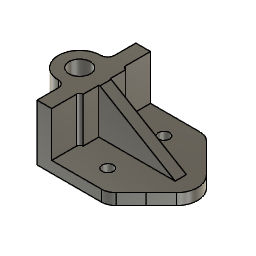
A3 (Autodesk Fusion 360 design; units mm, degrees)
Autodesk Fusion 360 part; units mm, degrees
sketch "BaseA3" plane through (0, 0, 0) normal (0, 0, 1) x (1, 0, 0)
  line L0 (0, 0) -> (28, 0)
  line L1 (28, 88) -> (0, 88)
  line L2 (0, 0) -> (-3, 0)
  line L3 (-3, 88) -> (0, 88)
  line L4 (-3, 0) -> (-16, 0)
  line L5 (-16, 88) -> (-3, 88)
  line L6 (-9.5, 0) -> (-9.5, 44) construction
  line L7 (-9.5, 44) -> (-16, 44) construction
  line L8 (-16, 44) -> (-22, 44) construction
  circle A0 centre (-22, 44) radius 9.5
  arc A1 (-22, 63) -> (-22, 25) centre (-22, 44) ccw
  line L9 (-16, 0) -> (-16, 19)
  line L10 (-16, 69) -> (-16, 88)
  arc A2 (-22, 63) -> (-16, 69) centre (-22, 69) ccw
  arc A3 (-16, 19) -> (-22, 25) centre (-22, 19) ccw
  line L11 (0, 63) -> (0, 63)
  line L12 (0, 25) -> (0, 22) construction
  line L13 (0, 22) -> (-3, 22) construction
  arc A4 (0, 25) -> (-3, 22) centre (0, 22) ccw
  line L14 (-9.5, 44) -> (0, 44) construction
  arc A5 (-3, 66) -> (0, 63) centre (0, 66) ccw
  line L15 (-22, 69) -> (-22, 63) construction
  line L16 (-22, 69) -> (-16, 69) construction
  line L17 (-22, 63) -> (-22, 25) construction
  line L18 (-22, 25) -> (-22, 19) construction
  line L19 (-22, 19) -> (-16, 19) construction
  line L20 (0, 63) -> (0, 66) construction
  line L21 (0, 66) -> (-3, 66) construction
  line L22 (-3, 69) -> (28, 69) construction
  circle A6 centre (28, 69) radius 5
  line L23 (0, 44) -> (28, 44) construction
  circle A7 centre (28, 19) radius 5
  line L24 (-3, 19) -> (28, 19) construction
  line L25 (28, 19) -> (64, 19) construction
  line L26 (64, 19) -> (64, 69) construction
  line L27 (64, 69) -> (28, 69) construction
  line L28 (28, 0) -> (46.834, 0)
  line L29 (46.834, 0) -> (64, 17.146)
  line L30 (64, 17.146) -> (77.427, 30.5569)
  line L31 (28, 44) -> (83, 44) construction
  line L32 (64, 70.854) -> (77.427, 57.4431)
  line L33 (46.834, 88) -> (64, 70.854)
  line L34 (28, 88) -> (46.834, 88)
  arc A8 (77.427, 30.5569) -> (77.427, 57.4431) centre (64, 44) ccw
  line L35 (-3, 88) -> (-3, 66)
  line L36 (-3, 22) -> (-3, 0)
  line L37 (-3, 0) -> (-3, 22)
  line L38 (-3, 66) -> (-3, 88)
  line L39 (0, 49) -> (1, 49)
  line L40 (1, 49) -> (1, 39)
  line L41 (1, 39) -> (0, 39)
  line L42 (0, 63) -> (0, 49)
  line L43 (0, 39) -> (0, 25)
  dimension "d3" = 13
  dimension "d4" = 88
  dimension "d5" = 19
  constraint coincident L0.start L2.start
  constraint horizontal L0
  constraint horizontal L1
  constraint horizontal L2
  constraint vertical L37
  constraint horizontal L3
  constraint vertical L42
  constraint horizontal L4
  constraint vertical L9
  constraint horizontal L5
  constraint vertical L35
  constraint midpoint L4 L6.start
  constraint perpendicular L4 L6
  constraint perpendicular L7 L9
  constraint perpendicular L8 L9
  constraint coincident L8.end A0.centre
  constraint concentric A0 A1
  constraint tangent A1 L35
  constraint collinear L9 L10
  constraint coincident L7.end L9
  constraint tangent L10 A2
  constraint symmetric L7 L10.start L9.end
  constraint symmetric L7 A1.start A1.end
  constraint symmetric L7 A2 A3
  constraint perpendicular L11 L42
  constraint coincident L13.end L35
  constraint perpendicular L13 L35
  constraint coincident L12.end L13.start
  constraint symmetric L12.start L14 L11.start
  constraint symmetric L13.end L14 A5.start
  constraint symmetric A4 L14 A5
  constraint coincident A2.centre L15.start
  constraint vertical L15
  constraint coincident A3.centre L18.end
  constraint coincident A5.centre L20.end
  constraint coincident L22.start L35
  constraint perpendicular L22 L35
  constraint coincident L22.end A6.centre
  constraint symmetric A6 L23 A7
  constraint symmetric L22.start L23 L24.start
  constraint symmetric L22.end L23 A7.centre
  constraint coincident A7.centre L24.end
  constraint perpendicular L25 L26
  constraint midpoint L26 A8.centre
  constraint tangent L30 A8
  constraint coincident L31.end A8
  constraint symmetric L0.end L31 L1.start
  constraint symmetric L29.end L31 L32.start
  constraint symmetric L28.end L31 L33.start
  constraint symmetric L30.end L31 L32.end
  constraint collinear L35 L36
  constraint collinear L37 L38
  constraint perpendicular L23 L40
  constraint coincident L41.end L42
  constraint perpendicular L41 L42
  constraint collinear L42 L43
  constraint coincident L14.end L42
  measures "d3" distance of L2.end L4.end
  measures "d4" distance of L2.end L3.start
  measures "d5" diameter of A0
extrude "Extrude1" add sketch "BaseA3" along normal blind 10 contours L0 L1 L2 L3 A4 A5 L28 L29 L30 L32 L33 L34 A8 L35 L36 L37 L38 L39 L40 L41 L42 L43
extrude "Extrude2" add sketch "BaseA3" along normal blind 50 contours L4 L5 A1 L9 L10 A2 A3 A4 A5 L35 L36 L37 L38 L39 L40 L41 L42 L43
fillet "Fillet1" radius 13 1 edges at (46.834, 0, 5)
fillet "Fillet2" radius 13 1 edges at (46.834, 88, 5)
sketch "Triangle" plane through (0, 0, 0) normal (0, -1, 0) x (1, 0, 0)
  line L0 (41.4537, 0) -> (41.4537, 10)
  line L1 (41.4537, 10) -> (-3, 10)
  line L2 (-3, 10) -> (-3, 50)
  line L3 (-3, 50) -> (-16, 50)
  line L4 (-16, 50) -> (-16, 0)
  line L5 (-16, 0) -> (41.4537, 0)
  line L6 (-3, 10) -> (1, 10)
  line L7 (1, 50) -> (1, 10)
  line L8 (1, 10) -> (68, 10)
  line L9 (68, 10) -> (1, 50)
  constraint coincident L1.end L2.start
  constraint coincident L1 L6.end
  constraint perpendicular L2 L6
  constraint perpendicular L6 L7
  constraint perpendicular L7 L8
extrude "Extrude3" add sketch "Triangle" against normal blind 10 from surface at -39 contours L1 L7 L8 L9
named bodies: "MainBodyA3"
